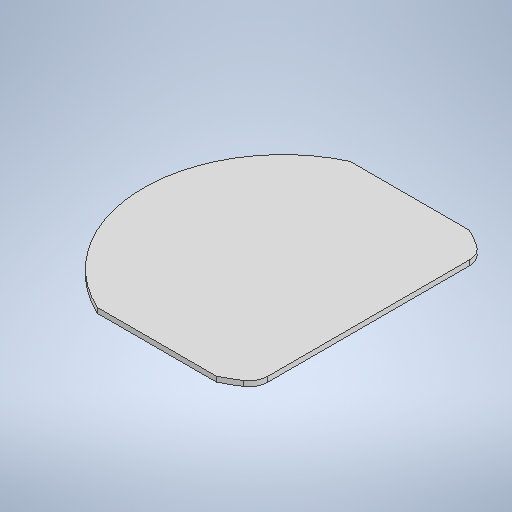
# Autodesk Inventor part: tapa_carcasa_4.0
Saved by Autodesk Inventor 2025.3 (Build 293356030, 356C)
## iProperties
Created: 2025-10-09
Part Number: tapa_carcasa_4.0
Material: Generic
Document SubType Name: Modeling
Designer: brene
Density: 1 g/cm^3
Appearance: Default
Author: brene
Autodesk Inventor part; units mm, degrees
ref_plane "YZ Plane" through (0, 0, 0) normal (1, 0, 0) x (0, 1, 0)
ref_plane "XZ Plane" through (0, 0, 0) normal (0, 1, 0) x (-1, 0, 0)
ref_plane "XY Plane" through (0, 0, 0) normal (0, 0, 1) x (1, 0, 0)
sketch "Sketch3" plane through (0, 0, 0) normal (0, 1, 0) x (-1, 0, 0)
  line L0 (-73.5, 0) -> (-68.4616, 0)
  line L1 (-68.4616, 0) -> (73.5, 0) construction
  line L2 (0, 0) -> (0, 66.5)
  line L3 (0, 66.5) -> (-31.305, 66.5)
  line L4 (0, 66.5) -> (31.305, 66.5)
  line L5 (0, 0) -> (0, -66.5)
  line L6 (0, -66.5) -> (31.305, -66.5)
  line L7 (0, -66.5) -> (-31.305, -66.5)
  arc A0 (31.305, -66.5) -> (31.305, 66.5) centre (0, 0) ccw
  line L8 (0, 0) -> (-45, 0)
  line L9 (-45, 0) -> (-45, 52.9835)
  line L10 (-45, 0) -> (-45, -52.9835)
  arc A1 (-31.305, 66.5) -> (-40.5118, 61.3273) centre (0, 0) ccw
  arc A2 (-40.5118, -61.3273) -> (-31.305, -66.5) centre (0, 0) ccw
  arc A3 (-40.5118, 61.3273) -> (-45, 52.9835) centre (-35, 52.9835) ccw
  arc A4 (-45, -52.9835) -> (-40.5118, -61.3273) centre (-35, -52.9835) ccw
  point P0 (-45, 58.1141)
  point P1 (-45, -58.1141)
  dimension "d13" = 66.5
  dimension "d14" = 66.5
  dimension "d16" = 73.5
  dimension "d17" = 73.5
  dimension "d18" = 58.1141
  dimension "d19" = 58.1141
  dimension "d20" = 10
  dimension "d21" = 10
  dimension "d24" = 45
  constraints: 22 end point, 13 point on circle, 5 centre point, 4 point on line, 4 tangent, 3 horizontal, 3 vertical, 2 perpendicular, 1 coincident, 1 parallel
  measures "d13" distance of L2.start L2.end
  measures "d14" distance of L2.start L5.end
  measures "d16" radius of A0
  measures "d17" radius of A2
  measures "d18" distance of L8.end point (-45, 58.114)
  measures "d19" distance of L8.end point (-45, -58.114)
  measures "d20" radius of A3
  measures "d21" radius of A4
  measures "d24" distance of L2.start L8.end
extrude "Extrusion2" add sketch "Sketch3" along normal blind 2.7
body "Solid2"
